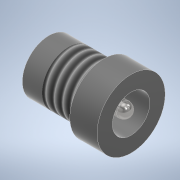
# Autodesk Inventor part: DC Jack
Saved by Autodesk Inventor 2022 (Build 260153000, 153)
## iProperties
Created: 2022-06-10
Part Number: DC Jack
Material: Generic
Document SubType Name: Modeling
Designer: Nick
Density: 1 g/cm^3
Appearance: Smooth - Black
Author: Nick
Autodesk Inventor part; units mm, degrees
ref_plane "YZ Plane" through (0, 0, 0) normal (1, 0, 0) x (0, 1, 0)
ref_plane "XZ Plane" through (0, 0, 0) normal (0, 1, 0) x (-1, 0, 0)
ref_plane "XY Plane" through (0, 0, 0) normal (0, 0, 1) x (1, 0, 0)
sketch "Sketch1" plane through (0, 0, 0) normal (0, 0, 1) x (1, 0, 0)
  line L0 (0, 0) -> (12.07, 0)
  line L1 (12.07, 0) -> (12.07, 5)
  line L2 (12.07, 5) -> (8.07, 5)
  line L3 (8.07, 5) -> (8.07, 3.9)
  line L4 (8.07, 3.9) -> (0, 3.9)
  line L5 (0, 3.9) -> (0, 0)
  dimension "d0" = 7.8
  dimension "d1" = 8.07
  dimension "d2" = 4
  dimension "d3" = 10
  constraints: 12 end point, 4 perpendicular, 1 horizontal, 1 vertical
  measures "d0" diameter of L4 L0
  measures "d1" distance of L3.end L4.end
  measures "d2" distance of L1.end L2.end
  measures "d3" diameter of L2 L0
revolve "Revolution1" add sketch "Sketch1" angle 360 about axis through (0, 0, 0) along (1, 0, 0)
thread "Thread1" size "M8x1.25" class "6g" standard "ANSI Metric M Profile" length 5.17 offset 2.9
sketch "Sketch2" plane through (12.07, 0, 0) normal (1, 0, 0) x (0, 0, -1)
  circle A0 centre (0, 0) radius 2.75
  circle A1 centre (0, 0) radius 1.05
  dimension "d7" = 5.5
  dimension "d8" = 2.1
  constraints: 2 centre point, 2 coincident
  measures "d7" diameter of A0
  measures "d8" diameter of A1
extrude "Extrusion1" cut sketch "Sketch2" against normal blind 4
fillet "Fillet1" radius 1.05 1 edges at (12.07, 0, 1.05)
body "Solid1"
